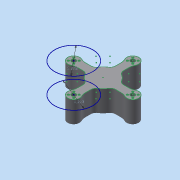
# Autodesk Inventor part: outline
Saved by Autodesk Inventor 2015 (Build 190159000, 159)
## iProperties
Created: 2016-01-29
Part Number: outline
Material: Generic
Document SubType Name: Modeling
Designer: Raphael
Density: 1 g/cm^3
Appearance: Default
Author: Raphael
Autodesk Inventor part; units mm, degrees
ref_plane "YZ Plane" through (0, 0, 0) normal (1, 0, 0) x (0, 1, 0)
ref_plane "XZ Plane" through (0, 0, 0) normal (0, 1, 0) x (-1, 0, 0)
ref_plane "XY Plane" through (0, 0, 0) normal (0, 0, 1) x (1, 0, 0)
sketch "Sketch1" plane through (0, 0, 0) normal (0, 1, 0) x (-1, 0, 0)
  line L0 (15.1438, 4.7625) -> (29.7948, 4.7625)
  line L1 (29.7948, -4.7625) -> (15.1438, -4.7625)
  line L2 (68.405, 0) -> (-52.905, 0) projected
  line L3 (0, -52.905) -> (0, 68.405) projected
  line L4 (-4.7625, 15.1438) -> (-4.7625, 29.7948)
  line L5 (4.7625, 29.7948) -> (4.7625, 15.1438)
  line L6 (-15.1438, -4.7625) -> (-29.7948, -4.7625)
  line L7 (-29.7948, 4.7625) -> (-15.1438, 4.7625)
  line L8 (4.7625, -15.1438) -> (4.7625, -29.7948)
  line L9 (-4.7625, -29.7948) -> (-4.7625, -15.1438)
  arc A0 (-4.7625, 15.1438) -> (-15.1438, 4.7625) centre (0, 0) ccw
  arc A1 (-15.1438, -4.7625) -> (-4.7625, -15.1438) centre (0, 0) ccw
  arc A2 (4.7625, -15.1438) -> (15.1438, -4.7625) centre (0, 0) ccw
  arc A3 (15.1438, 4.7625) -> (4.7625, 15.1438) centre (0, 0) ccw
  arc A4 (-29.7948, 4.7625) -> (-29.7948, -4.7625) centre (-34.925, 0) ccw
  arc A5 (4.7625, 29.7948) -> (-4.7625, 29.7948) centre (0, 34.925) ccw
  arc A6 (29.7948, -4.7625) -> (29.7948, 4.7625) centre (34.925, 0) ccw
  arc A7 (-4.7625, -29.7948) -> (4.7625, -29.7948) centre (0, -34.925) ccw
  dimension "d9" = 9.525
  dimension "d12" = 360
  dimension "d14" = 15.875
  dimension "d17" = 30.1625
  dimension "d18" = 30.1625
  dimension "d19" = 30.1625
  dimension "d20" = 30.1625
  dimension "d21" = 14
  constraints: 16 end point, 16 point on circle, 8 centre point, 3 point on line, 1 coincident, 1 horizontal, 1 parallel, 26 other
  measures "d9" distance between parallel lines of L0 L1
  measures "d14" radius of A1
  measures "d21" diameter of A5
extrude "Extrusion1" add sketch "Sketch1" along normal blind 25.4
fillet "Fillet1" radius 6.35 8 edges at (4.7625, 12.7, 15.1438) (15.1438, 12.7, 4.7625) (15.1438, 12.7, -4.7625) (4.7625, 12.7, -15.1438) (-4.7625, 12.7, -15.1438) (-15.1438, 12.7, -4.7625) (-15.1438, 12.7, 4.7625) (-4.7625, 12.7, 15.1438)
fillet "Fillet1" radius 12.7 8 edges at (29.7948, 12.7, 4.7625) (29.7948, 12.7, -4.7625) (4.7625, 12.7, -29.7948) (-4.7625, 12.7, -29.7948) (-29.7948, 12.7, -4.7625) (-29.7948, 12.7, 4.7625) (-4.7625, 12.7, 29.7948) (4.7625, 12.7, 29.7948)
sketch "Sketch2" plane through (0, 25.4, 0) normal (0, 1, 0) x (1, 0, 0)
  arc A0 (6.2049, 31.6848) -> (-6.2049, 31.6848) centre (0, 34.925) ccw projected
  circle A1 centre (-3.182, 38.107) radius 1.1
  circle A2 centre (3.182, 38.107) radius 1.1
  circle A3 centre (3.182, 31.743) radius 1.1
  circle A4 centre (-3.182, 31.743) radius 1.1
  line L0 (3.182, 38.107) -> (-3.182, 31.743)
  line L1 (3.182, 31.743) -> (-3.182, 38.107)
  circle A5 centre (0, 34.925) radius 2.54
  point P0 (0, 0)
  dimension "d26" = 2.2
  dimension "d27" = 2.2
  dimension "d28" = 2.2
  dimension "d29" = 2.2
  dimension "d30" = 9
  dimension "d31" = 9
  dimension "d32" = 5.08
  constraints: 5 centre point, 4 end point, 4 midpoint, 1 coincident, 1 horizontal alignment, 1 perpendicular
  measures "d26" diameter of A1
  measures "d27" diameter of A2
  measures "d28" diameter of A3
  measures "d29" diameter of A4
  measures "d30" distance of L1.start L1.end
  measures "d31" distance of L0.start L0.end
  measures "d32" diameter of A5
extrude "Extrusion2" cut sketch "Sketch2" against normal through all
pattern_circular "Circular Pattern1" count 4 over 360 about axis through (0, -10, 0) along (0, 1, 0) of "Extrusion2"
sketch "Sketch3" plane through (0, 25.4, 0) normal (0, 1, 0) x (1, 0, 0)
  circle A0 centre (-34.925, 0) radius 2.54 projected
  circle A1 centre (0, 34.925) radius 2.54 projected
  circle A2 centre (31.743, 3.182) radius 1.1 projected
  circle A3 centre (34.925, 0) radius 2.54 projected
  circle A4 centre (31.743, -3.182) radius 1.1 projected
  circle A5 centre (38.107, 3.182) radius 1.1 projected
  circle A6 centre (38.107, -3.182) radius 1.1 projected
  circle A7 centre (3.182, -31.743) radius 1.1 projected
  circle A8 centre (0, -34.925) radius 2.54 projected
  circle A9 centre (-3.182, -31.743) radius 1.1 projected
  circle A10 centre (3.182, -38.107) radius 1.1 projected
  circle A11 centre (-3.182, -38.107) radius 1.1 projected
  circle A12 centre (-31.743, -3.182) radius 1.1 projected
  circle A13 centre (-34.925, 0) radius 2.54 projected
  circle A14 centre (-31.743, 3.182) radius 1.1 projected
  circle A15 centre (-38.107, -3.182) radius 1.1 projected
  circle A16 centre (-38.107, 3.182) radius 1.1 projected
  circle A17 centre (-3.182, 31.743) radius 1.1 projected
  circle A18 centre (3.182, 38.107) radius 1.1 projected
  circle A19 centre (-3.182, 38.107) radius 1.1 projected
  circle A20 centre (3.182, 31.743) radius 1.1 projected
  circle A21 centre (0, 34.925) radius 2.54 projected
  arc A22 (-13.7482, -7.9375) -> (-7.9375, -13.7482) centre (0, 0) ccw projected
  arc A23 (-6.2049, -31.6848) -> (-4.7625, -25.8063) centre (-17.4625, -25.8063) ccw projected
  arc A24 (-6.2049, -31.6848) -> (6.2049, -31.6848) centre (0, -34.925) ccw projected
  arc A25 (4.7625, -25.8063) -> (6.2049, -31.6848) centre (17.4625, -25.8063) ccw projected
  arc A26 (7.9375, -13.7482) -> (13.7482, -7.9375) centre (0, 0) ccw projected
  arc A27 (31.6848, -6.2049) -> (25.8063, -4.7625) centre (25.8063, -17.4625) ccw projected
  arc A28 (31.6848, -6.2049) -> (31.6848, 6.2049) centre (34.925, 0) ccw projected
  arc A29 (25.8063, 4.7625) -> (31.6848, 6.2049) centre (25.8063, 17.4625) ccw projected
  arc A30 (13.7482, 7.9375) -> (7.9375, 13.7482) centre (0, 0) ccw projected
  arc A31 (6.2049, 31.6848) -> (4.7625, 25.8063) centre (17.4625, 25.8063) ccw projected
  arc A32 (6.2049, 31.6848) -> (-6.2049, 31.6848) centre (0, 34.925) ccw projected
  arc A33 (-4.7625, 25.8063) -> (-6.2049, 31.6848) centre (-17.4625, 25.8063) ccw projected
  arc A34 (-7.9375, 13.7482) -> (-13.7482, 7.9375) centre (0, 0) ccw projected
  arc A35 (-31.6848, 6.2049) -> (-25.8063, 4.7625) centre (-25.8063, 17.4625) ccw projected
  arc A36 (-31.6848, 6.2049) -> (-31.6848, -6.2049) centre (-34.925, 0) ccw projected
  arc A37 (-25.8063, -4.7625) -> (-31.6848, -6.2049) centre (-25.8063, -17.4625) ccw projected
  circle A38 centre (-34.925, 0) radius 22.5
  circle A39 centre (0, -34.925) radius 22.5
  line L0 (-25.8063, -4.7625) -> (-19.2474, -4.7625) projected
  arc A40 (-13.7482, -7.9375) -> (-19.2474, -4.7625) centre (-19.2474, -11.1125) ccw projected
  arc A41 (-4.7625, -19.2474) -> (-7.9375, -13.7482) centre (-11.1125, -19.2474) ccw projected
  line L1 (-4.7625, -19.2474) -> (-4.7625, -25.8063) projected
  line L2 (4.7625, -25.8063) -> (4.7625, -19.2474) projected
  arc A42 (7.9375, -13.7482) -> (4.7625, -19.2474) centre (11.1125, -19.2474) ccw projected
  arc A43 (19.2474, -4.7625) -> (13.7482, -7.9375) centre (19.2474, -11.1125) ccw projected
  line L3 (19.2474, -4.7625) -> (25.8063, -4.7625) projected
  line L4 (25.8063, 4.7625) -> (19.2474, 4.7625) projected
  arc A44 (13.7482, 7.9375) -> (19.2474, 4.7625) centre (19.2474, 11.1125) ccw projected
  arc A45 (4.7625, 19.2474) -> (7.9375, 13.7482) centre (11.1125, 19.2474) ccw projected
  line L5 (4.7625, 19.2474) -> (4.7625, 25.8063) projected
  line L6 (-4.7625, 25.8063) -> (-4.7625, 19.2474) projected
  arc A46 (-7.9375, 13.7482) -> (-4.7625, 19.2474) centre (-11.1125, 19.2474) ccw projected
  arc A47 (-19.2474, 4.7625) -> (-13.7482, 7.9375) centre (-19.2474, 11.1125) ccw projected
  line L7 (-19.2474, 4.7625) -> (-25.8063, 4.7625) projected
  point P0 (0, 0)
  dimension "d38" = 45
  dimension "d39" = 45
  constraints: 2 centre point, 2 coincident
  measures "d38" diameter of A38
  measures "d39" diameter of A39
equation "\"d17\" = arm"
equation "\"d18\" = arm"
equation "\"d19\" = arm"
equation "\"d20\" = arm"
equation "\"arm\" = 30.1625"
body "Solid1"
